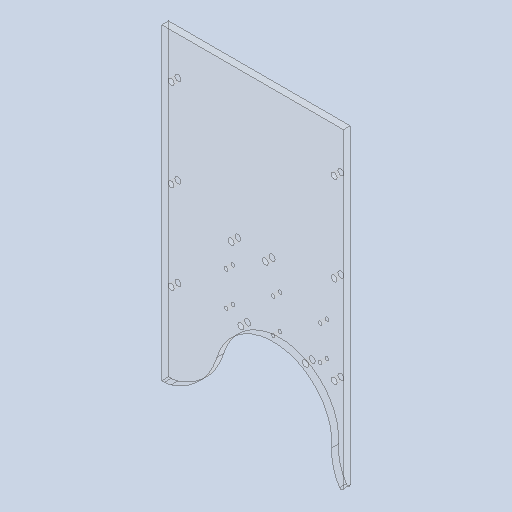
# Autodesk Inventor part: Lower Deck
Saved by Autodesk Inventor 2022 (Build 260153000, 153)
## iProperties
Created: 2022-10-14
Part Number: Lower Deck
Material: Polycarbonate, Clear
Document SubType Name: Modeling
Designer: matt
Density: 1.2 g/cm^3
Appearance: Polycarbonate - Clear
Mass: 323.479 g
Surface Area: 921.566 cm^2
Volume: 269.566 cm^3
Author: matt
Autodesk Inventor part; units mm, degrees
ref_plane "YZ Plane" through (0, 0, 0) normal (1, 0, 0) x (0, 1, 0)
ref_plane "XZ Plane" through (0, 0, 0) normal (0, 1, 0) x (-1, 0, 0)
ref_plane "XY Plane" through (0, 0, 0) normal (0, 0, 1) x (1, 0, 0)
sketch "Sketch1" plane through (0, 0, 0) normal (0, 0, 1) x (1, 0, 0)
  line L0 (177.0985, -0.0099) -> (177.0985, 299.9901)
  line L1 (177.0985, 299.9901) -> (-0.7015, 299.9901) construction
  line L2 (-0.7015, 299.9901) -> (-0.7015, 12.8831)
  line L3 (3.1985, 12.8831) -> (5.7502, 12.8831)
  arc A0 (162.2875, 38.1203) -> (54.7536, 57.5761) centre (107.4018, 41.6649) ccw
  arc A1 (11.9285, 13.8613) -> (54.7536, 57.5761) centre (-8.4768, 76.6855) ccw
  arc A2 (5.7502, 12.8831) -> (11.9285, 13.8613) centre (5.7502, 32.8831) ccw
  circle A3 centre (164.4485, 93.4388) radius 2.8
  circle A4 centre (164.4485, 176.4531) radius 2.8
  circle A5 centre (164.4485, 259.4675) radius 2.8
  circle A6 centre (11.9485, 259.4675) radius 2.8
  circle A7 centre (11.9485, 176.4531) radius 2.8
  circle A8 centre (11.9485, 93.4388) radius 2.8
  arc A9 (162.2875, 38.1203) -> (169.4999, 9.3715) centre (210.7223, 34.9923) ccw
  line L4 (83.4018, 393.7) -> (83.4018, -22.225) construction
  line L5 (83.4018, -22.225) -> (131.4018, -22.225) construction
  line L6 (131.4018, -22.225) -> (131.4018, 393.7) construction
  line L7 (131.4018, 393.7) -> (83.4018, 393.7) construction
  line L8 (83.4018, 393.7) -> (131.4018, -22.225) construction
  line L9 (83.4018, -22.225) -> (131.4018, 393.7) construction
  line L10 (36.4143, 133.6649) -> (149.1268, 133.6649) construction
  line L11 (41.1768, 101.6649) -> (144.3643, 101.6649) construction
  circle A10 centre (63.4018, 133.6649) radius 1.75
  circle A11 centre (63.4018, 101.6649) radius 1.75
  line L12 (63.4018, 133.6649) -> (63.4018, 101.6649) construction
  line L13 (107.4018, 31.6649) -> (107.4018, 185.7375) construction
  circle A12 centre (107.4018, 133.6649) radius 1.75
  circle A13 centre (107.4018, 101.6649) radius 1.75
  circle A14 centre (151.4018, 133.6649) radius 1.75
  circle A15 centre (151.4018, 101.6649) radius 1.75
  line L14 (151.4018, 133.6649) -> (151.4018, 101.6649) construction
  line L15 (173.1985, 301.3071) -> (173.1985, 10.4273)
  line L16 (177.0985, -0.0099) -> (177.0985, 42.269)
  line L17 (3.1985, 301.3071) -> (3.1985, 12.8831)
  line L18 (-0.7015, 12.8831) -> (-0.7015, 42.269)
  line L19 (24.0985, 301.3071) -> (-0.2015, 301.3071) projected
  line L20 (3.1985, 301.3071) -> (173.1985, 301.3071)
  line L21 (177.0985, 301.3071) -> (177.0985, 299.9901)
  line L22 (177.0985, 299.9901) -> (-0.7015, 299.9901) construction
  line L23 (-0.7015, 299.9901) -> (-0.7015, 301.3071)
  circle A16 centre (107.4018, 41.6649) radius 50.5415 projected
  circle A17 centre (137.6518, 94.0594) radius 2.8
  line L24 (137.6518, 94.0594) -> (107.4018, 41.6649) construction
  line L25 (107.4018, 41.6649) -> (75.7506, 96.4865) construction
  circle A18 centre (77.1518, 94.0594) radius 2.8
  arc A19 (169.4999, 9.3715) -> (173.1985, 10.4273) centre (171.1985, 10.4273) ccw
  circle A20 centre (100.0728, 157.9036) radius 4.75 projected
  circle A21 centre (68.0733, 158.0877) radius 4.75 projected
  circle A22 centre (100.0728, 157.9036) radius 2.8
  circle A23 centre (68.0733, 158.0877) radius 2.8
  point P0 (0, 0)
  point P1 (152.4018, -0.0099)
  point P2 (173.1985, 42.269)
  point P3 (3.1985, 42.269)
  point P4 (174.0985, 3.1425)
  point P5 (24.0985, 301.3071)
  point P6 (173.1985, 4.2079)
  dimension "d0" = 177.8
  dimension "d1" = 300
  dimension "d9" = 258.3252
  dimension "d10" = 55
  dimension "d11" = 108.1033
  dimension "d12" = 48
  dimension "d13" = 32
  dimension "d14" = 3.5
  dimension "d15" = 3.5
  dimension "d16" = 20
  dimension "d17" = 3.5
  dimension "d18" = 3.5
  dimension "d19" = 3.5
  dimension "d20" = 3.5
  dimension "d21" = 20
  dimension "d22" = 3.9
  dimension "d23" = 3.9
  dimension "d24" = 60
  dimension "d25" = 5.6
  dimension "d26" = 60.5
  dimension "d27" = 60
  dimension "d28" = 60
  dimension "d29" = 5.6
  dimension "d30" = 60.5
  dimension "d31" = 2
  dimension "d32" = 5.6
  dimension "d33" = 5.6
  constraints: 50 end point, 21 centre point, 14 point on line, 11 point on circle, 9 parallel, 6 perpendicular, 6 tangent, 4 midpoint, 3 horizontal, 2 coincident, 1 vertical
  measures "d0" distance of L1.end L0.end
  measures "d1" distance of L0.end L0.start
  measures "d9" distance from line of L1 A0.centre
  measures "d10" radius of A0
  measures "d11" distance from line of A0.centre L2
  measures "d12" distance of L5.end L4.end
  measures "d13" distance between parallel lines of L11 L10
  measures "d14" diameter of A10
  measures "d15" diameter of A11
  measures "d16" distance between parallel lines of L4 L12
  measures "d17" diameter of A12
  measures "d18" diameter of A13
  measures "d19" diameter of A14
  measures "d20" diameter of A15
  measures "d21" distance between parallel lines of L14 L6
  measures "d22" distance between parallel lines of L15 L0
  measures "d23" distance between parallel lines of L2 L17
  measures "d24" distance from line of A0.centre L11
  measures "d25" diameter of A17
  measures "d26" distance of A0.centre L24.start
  measures "d27" angle of L24 L11
  measures "d28" angle of L25 L24
  measures "d29" diameter of A18
  measures "d30" distance of A0.centre A18.centre
  measures "d31" radius of A19
  measures "d32" diameter of A22
  measures "d33" diameter of A23
extrude "Extrusion1" add sketch "Sketch1" along normal blind 6.35 contours L17 L19 L20 L15 A19 A9 A0 A1 A2 L3 | A20 | A21
equation "\"d21\" = d16"
equation "\"d30\" = d26"
body "Solid1"
